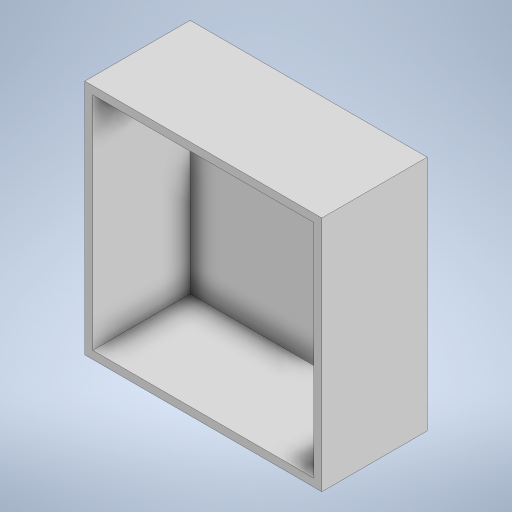
# Autodesk Inventor part: Temp_controller_box
Saved by Autodesk Inventor 2024 (Build 280153000, 153)
## iProperties
Created: 2026-04-14
Part Number: Temp_controller_box
Material: Generic
Document SubType Name: Modeling
Designer: Péter
Density: 1 g/cm^3
Appearance: Default
Author: Péter
Autodesk Inventor part; units mm, degrees
ref_plane "YZ Plane" through (0, 0, 0) normal (1, 0, 0) x (0, 1, 0)
ref_plane "XZ Plane" through (0, 0, 0) normal (0, 1, 0) x (-1, 0, 0)
ref_plane "XY Plane" through (0, 0, 0) normal (0, 0, 1) x (1, 0, 0)
sketch "Sketch1" plane through (0, 0, 0) normal (0, 0, 1) x (1, 0, 0)
  line L0 (-45, 45) -> (45, 45)
  line L1 (45, 45) -> (45, -45)
  line L2 (45, -45) -> (-45, -45)
  line L3 (-45, -45) -> (-45, 45)
  line L4 (-45, 45) -> (45, -45) construction
  line L5 (45, 45) -> (-45, -45) construction
  point P0 (0, 0)
  dimension "d0" = 90
  dimension "d1" = 90
  constraints: 12 end point, 2 midpoint, 2 parallel, 1 horizontal, 1 perpendicular
  measures "d0" distance of L1.end L2.end
  measures "d1" distance of L0.end L1.end
extrude "Extrusion1" add sketch "Sketch1" along normal blind 40
shell "Shell1" thickness 3 removed faces 1 at (-15, 15, 40)
body "Solid1"
